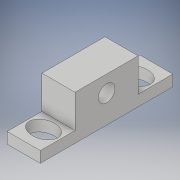
# Autodesk Inventor part: SuperiorBancada
Saved by Autodesk Inventor 2019 (Build 230136000, 136)
## iProperties
Created: 2019-07-02
Part Number: SuperiorBancada
Material: Generic
Document SubType Name: Modeling
Designer: Oscar Rojas
Density: 1 g/cm^3
Appearance: Default
Mass: 9.25971 g
Surface Area: 40.8039 cm^2
Volume: 9.25971 cm^3
Author: Oscar Rojas
Autodesk Inventor part; units mm, degrees
ref_plane "YZ Plane" through (0, 0, 0) normal (1, 0, 0) x (0, 1, 0)
ref_plane "XZ Plane" through (0, 0, 0) normal (0, 1, 0) x (-1, 0, 0)
ref_plane "XY Plane" through (0, 0, 0) normal (0, 0, 1) x (1, 0, 0)
sketch "Sketch1" plane through (0, 0, 0) normal (0, 1, 0) x (-1, 0, 0)
  line L0 (0, 0) -> (-20, 0)
  line L1 (-20, 0) -> (-20, -60)
  line L2 (-20, -60) -> (0, -60)
  line L3 (0, -60) -> (0, 0)
  line L4 (0, -60) -> (-15, -60)
  line L5 (0, -60) -> (15, -60) construction
  line L6 (-15, -60) -> (-15, 0)
  dimension "d0" = 20
  dimension "d1" = 60
  dimension "d14" = 15
  dimension "d15" = 180
  constraints: 14 end point, 2 collinear, 2 horizontal, 2 parallel, 2 perpendicular, 1 point on line
  measures "d0" distance of L2.end L1.end
  measures "d1" distance of L1.end L0.end
  measures "d14" distance of L2.end L4.end
  measures "d15" angle of L4 L5
extrude "Extrusion1" add sketch "Sketch1" along normal blind 5
sketch "Sketch2" plane through (0, 5, 0) normal (0, 1, 0) x (1, 0, 0)
  line L0 (0, 0) -> (20, 0)
  line L1 (10, 0) -> (19, 0) construction
  line L2 (20, 60) -> (0, 60)
  line L3 (0, 60) -> (0, 0)
  line L4 (0, 30) -> (2.0385, 30)
  line L5 (0, 0) -> (15, 0)
  line L6 (0, 0) -> (20, 0) projected
  line L7 (0, 0) -> (15, 0) construction
  line L8 (7.5, 0) -> (16.5, 0) construction
  ellipse E0 centre (7.5, 9) end of major axis (1.0192, 9) minor radius 4.9353
  ellipse E1 centre (7.5, 51) end of major axis (1.0192, 51) minor radius 4.9353
  line L9 (0, 9) -> (1.0192, 9)
  constraints: 18 end point, 6 horizontal, 3 midpoint, 2 collinear, 1 horizontal alignment, 1 point on line, 1 symmetric about line, 4 other
sketch "Sketch3" plane through (0, 5, 0) normal (0, 1, 0) x (1, 0, 0)
  line L0 (0, 60) -> (0, 0) projected
  line L1 (20, 0) -> (20, 60) projected
  line L2 (0, 15.7197) -> (20, 15.7197)
  line L3 (20, 15.7197) -> (20, 44.2851)
  line L4 (20, 44.2851) -> (0, 44.2851)
  line L5 (0, 44.2851) -> (0, 15.7197)
  constraints: 8 end point, 2 parallel, 2 point on line, 1 horizontal, 1 perpendicular
extrude "Extrusion3" add sketch "Sketch3" along normal blind 15
sketch "Sketch4" plane through (20, 0, 0) normal (1, 0, 0) x (0, 0, -1)
  line L0 (15.7197, 5) -> (15.7197, 20) projected
  line L1 (44.2851, 5) -> (60, 5) projected
  circle A0 centre (30.0024, 12.5) radius 3.75
  point P0 (0, 0)
  dimension "d11" = 7.5
  constraints: 1 centre point
  measures "d11" diameter of A0
extrude "Extrusion4" cut sketch "Sketch4" against normal blind 65.5
extrude "Extrusion5" add sketch "Sketch1" along normal blind 5 contours L3 L2 L6 L0
extrude "Extrusion6" cut sketch "Sketch1" along normal blind 22.5 contours L6 L2 L1 L0
extrude "Extrusion8" cut sketch "Sketch2" against normal blind 26
body "Solid1"
